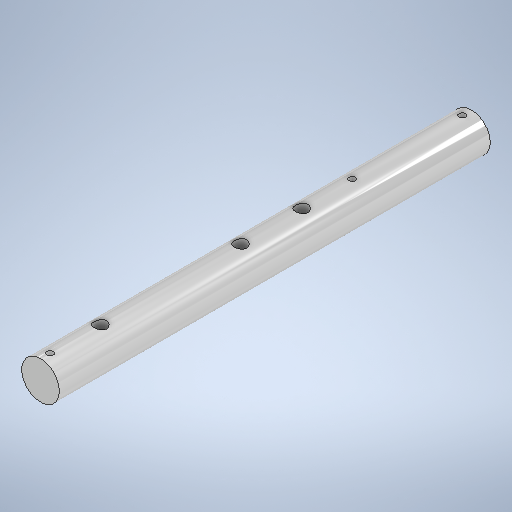
# Autodesk Inventor part: small_bar_roller
Saved by Autodesk Inventor 2025.1 (Build 291241000, 241)
## iProperties
Created: 2022-02-06
Part Number: small_bar_roller
Material: アルミニウム 6061-AHC
Document SubType Name: Modeling
Designer: 中島 青蔵
Density: 2.7 g/cm^3
Appearance: アルミニウム - ダーク
Author: 中島 青蔵
Autodesk Inventor part; units mm, degrees
ref_plane "YZ Plane" through (0, 0, 0) normal (1, 0, 0) x (0, 1, 0)
ref_plane "XY Plane" through (0, 0, 0) normal (0, 0, 1) x (1, 0, 0)
sketch "スケッチ1" plane through (0, 0, 0) normal (0, 0, 1) x (1, 0, 0)
  circle A0 centre (0, 0) radius 6
  dimension "d0" = 12
  constraints: 1 centre point, 1 coincident
  measures "d0" diameter of A0
extrude "押し出し1" add sketch "スケッチ1" along normal blind 137
ref_plane "作業平面1" through (0, 6, 0) normal (0, 1, 0) x (-1, 0, 0)
sketch "スケッチ2" plane through (0, 6, 0) normal (0, 1, 0) x (-1, 0, 0)
  line L0 (6, 0) -> (-6, 0) projected
  line L1 (6, 137) -> (-6, 137) projected
  point P0 (0, 0)
  point P1 (0, 3)
  point P2 (0, 134)
  point P3 (0, 118)
  point P4 (0, 38)
  point P5 (0, 73.5)
  point P6 (0, 54)
  dimension "d3" = 3
  dimension "d19" = 3
  dimension "d20" = 19
  dimension "d22" = 99
  dimension "d23" = 44.5
  dimension "d24" = 19.5
  measures "d3" distance from line of L0 point (0, 3)
  measures "d19" distance from line of L1 point (0, 134)
  measures "d20" distance from line of L1 point (0, 118)
  measures "d22" distance from line of L1 point (0, 38)
  measures "d23" distance of point (0, 118) point (0, 73.5)
  measures "d24" distance of point (0, 73.5) point (0, 54)
hole "穴1" at (0, 6, 3) at (0, 6, 134) at (0, 6, 38) direction (0, -1, 0) diameter 2 end through all
hole "穴2" at (0, 6, 118) at (0, 6, 73.5) at (0, 6, 54) direction (0, -1, 0) diameter 4 end through all
